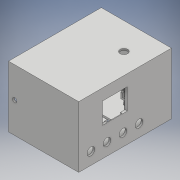
# Autodesk Inventor part: Suporte
Saved by Autodesk Inventor 2018 (Build 220112000, 112)
## iProperties
Created: 2018-04-23
Part Number: Suporte
Material: Genérico
Document SubType Name: Modeling
Designer: mirre
Density: 1 g/cm^3
Appearance: Padrão
Author: mirre
Autodesk Inventor part; units mm, degrees
sketch "Esboço1" plane through (0, 0, 0) normal (0, 0, 1) x (1, 0, 0)
  line L0 (0, 0) -> (118, 0)
  line L1 (118, 0) -> (118, 156)
  line L2 (118, 156) -> (0, 156)
  line L3 (0, 156) -> (0, 0)
  dimension "d0" = 118
  dimension "d1" = 156
  constraints: 8 end point, 2 parallel, 1 horizontal, 1 perpendicular
  measures "d0" distance of L2.end L1.end
  measures "d1" distance of L2.end L0.start
extrude "Extrusão1" add sketch "Esboço1" along normal blind 3
sketch "Esboço2" plane through (0, 0, 3) normal (0, 0, 1) x (1, 0, 0)
  line L0 (3, 3) -> (115, 3)
  line L1 (115, 3) -> (115, 153)
  line L2 (115, 153) -> (3, 153)
  line L3 (3, 153) -> (3, 3)
  line L4 (0, 156) -> (0, 0) projected
  line L5 (118, 156) -> (0, 156) projected
  line L6 (0, 0) -> (118, 0) projected
  line L7 (118, 0) -> (118, 156) projected
  dimension "d4" = 3
  dimension "d5" = 3
  dimension "d6" = 3
  dimension "d7" = 3
  constraints: 8 end point, 2 parallel, 1 horizontal, 1 perpendicular
  measures "d4" distance between parallel lines of L3 L4
  measures "d5" distance between parallel lines of L5 L2
  measures "d6" distance between parallel lines of L6 L0
  measures "d7" distance between parallel lines of L7 L1
extrude "Extrusão2" add sketch "Esboço2" along normal blind 100
sketch "Esboço3" plane through (0, 0, 3) normal (0, 0, 1) x (1, 0, 0)
  line L0 (3, 3) -> (3, 153) projected
  line L1 (3, 3) -> (8, 3)
  line L2 (8, 3) -> (8, 8)
  line L3 (8, 8) -> (3, 8)
  line L4 (3, 8) -> (3, 3)
  line L5 (115, 3) -> (3, 3) projected
  line L6 (68, 3) -> (73, 3)
  line L7 (73, 3) -> (73, 8)
  line L8 (73, 8) -> (68, 8)
  line L9 (68, 8) -> (68, 3)
  line L10 (3, 93) -> (8, 93)
  line L11 (8, 93) -> (8, 98)
  line L12 (8, 98) -> (3, 98)
  line L13 (3, 98) -> (3, 93)
  line L14 (68, 93) -> (73, 93)
  line L15 (73, 93) -> (73, 98)
  line L16 (73, 98) -> (68, 98)
  line L17 (68, 98) -> (68, 93)
  point P0 (0, 0)
  dimension "d10" = 5
  dimension "d11" = 5
  dimension "d12" = 5
  dimension "d13" = 5
  dimension "d14" = 95
  dimension "d15" = 70
  constraints: 32 end point, 8 parallel, 8 point on line, 4 horizontal, 4 perpendicular
  measures "d10" distance of L2.end L3.end
  measures "d11" distance of L7.end L8.end
  measures "d12" distance of L6.end L7.end
  measures "d13" distance of L14.end L15.end
  measures "d14" distance between parallel lines of L12 L1
  measures "d15" distance between parallel lines of L7 L0
extrude "Extrusão3" add sketch "Esboço3" along normal blind 5
sketch "Esboço4" plane through (0, 0, 3) normal (0, 0, 1) x (1, 0, 0)
  line L0 (115, 3) -> (3, 3) projected
  line L1 (3, 3) -> (3, 153) projected
  line L2 (3, 98) -> (23, 98)
  line L3 (23, 98) -> (23, 101)
  line L4 (23, 101) -> (3, 101)
  line L5 (3, 101) -> (3, 98)
  line L6 (73, 3) -> (76, 3)
  line L7 (76, 3) -> (76, 23)
  line L8 (76, 23) -> (73, 23)
  line L9 (73, 23) -> (73, 3)
  line L10 (73, 93) -> (73, 98) projected
  line L11 (73, 98) -> (73, 81)
  line L12 (73, 81) -> (76, 81)
  line L13 (76, 81) -> (76, 101)
  line L14 (76, 101) -> (56, 101)
  line L15 (56, 101) -> (56, 98)
  line L16 (73, 98) -> (68, 98) projected
  line L17 (56, 98) -> (73, 98)
  dimension "d197" = 3
  dimension "d198" = 3
  dimension "d199" = 3
  dimension "d200" = 3
  dimension "d201" = 20
  dimension "d202" = 20
  dimension "d203" = 20
  dimension "d204" = 20
  constraints: 28 end point, 6 perpendicular, 4 parallel, 2 horizontal, 1 collinear, 1 vertical
  measures "d197" distance between parallel lines of L7 L9
  measures "d198" distance between parallel lines of L13 L11
  measures "d199" distance between parallel lines of L14 L17
  measures "d200" distance between parallel lines of L2 L4
  measures "d201" distance between parallel lines of L5 L3
  measures "d202" distance between parallel lines of L13 L15
  measures "d203" distance between parallel lines of L12 L14
  measures "d204" distance between parallel lines of L0 L8
extrude "Extrusão4" add sketch "Esboço4" along normal blind 7
sketch "Esboço5" plane through (118, 0, 0) normal (1, 0, 0) x (0, 0, -1)
  circle A0 centre (-20.5, 20.5) radius 6
  circle A1 centre (-20.5, 47.5) radius 6
  circle A2 centre (-20.5, 74.5) radius 6
  circle A3 centre (-20.5, 101.5) radius 6
  line L0 (-83.5, 40.75) -> (-49, 40.75)
  line L1 (-49, 40.75) -> (-49, 81.25)
  line L2 (-49, 81.25) -> (-83.5, 81.25)
  line L3 (-83.5, 81.25) -> (-83.5, 40.75)
  line L4 (0, 0) -> (0, 156) projected
  line L5 (0, 0) -> (-103, 0) projected
  line L6 (-103, 0) -> (-103, 156) projected
  dimension "d48" = 12
  dimension "d50" = 12
  dimension "d52" = 12
  dimension "d54" = 12
  dimension "d58" = 27
  dimension "d59" = 27
  dimension "d60" = 27
  dimension "d61" = 40.5
  dimension "d62" = 34.5
  dimension "d68" = 20.5
  dimension "d72" = 28.5
  dimension "d73" = 28.5
  dimension "d74" = 28.5
  dimension "d75" = 28.5
  dimension "d76" = 20.5
  dimension "d77" = 20.25
  constraints: 8 end point, 4 centre point, 2 parallel, 1 horizontal, 1 perpendicular
  measures "d48" diameter of A0
  measures "d50" diameter of A1
  measures "d52" diameter of A2
  measures "d54" diameter of A3
  measures "d58" distance of A2.centre A1.centre
  measures "d59" distance of A3.centre A2.centre
  measures "d60" distance of A0.centre A1.centre
  measures "d61" distance between parallel lines of L2 L0
  measures "d62" distance between parallel lines of L1 L3
  measures "d68" distance from line of L5 A0.centre
  measures "d72" distance from line of L1 A0.centre
  measures "d73" distance from line of L1 A1.centre
  measures "d74" distance from line of L1 A2.centre
  measures "d75" distance from line of L1 A3.centre
  measures "d76" distance from line of L4 A3.centre
  measures "d77" distance from line of A3.centre L2
extrude "Extrusão5" cut sketch "Esboço5" against normal blind 20
sketch "Esboço6" plane through (115, 3, 3) normal (-1, 0, 0) x (0, 0, 1)
  line L0 (85.75, 79.5) -> (39.75, 79.5)
  line L1 (39.75, 79.5) -> (39.75, 36.5)
  line L2 (39.75, 36.5) -> (85.75, 36.5)
  line L3 (85.75, 36.5) -> (85.75, 79.5)
  line L4 (-3, -3) -> (100, -3) projected
  line L5 (-3, -3) -> (-3, 153) projected
  line L6 (88.75, 82.5) -> (36.75, 82.5)
  line L7 (36.75, 82.5) -> (36.75, 33.5)
  line L8 (36.75, 33.5) -> (88.75, 33.5)
  line L9 (88.75, 33.5) -> (88.75, 82.5)
  line L10 (46, 37.75) -> (80.5, 37.75) projected
  line L11 (80.5, 37.75) -> (80.5, 78.25) projected
  line L12 (100, -3) -> (100, 153) projected
  dimension "d82" = 1.25
  dimension "d83" = 5.25
  dimension "d84" = 49
  dimension "d85" = 52
  dimension "d88" = 3
  dimension "d89" = 3
  dimension "d90" = 3
  dimension "d91" = 3
  constraints: 16 end point, 4 parallel, 2 horizontal, 2 perpendicular
  measures "d82" distance between parallel lines of L2 L10
  measures "d83" distance between parallel lines of L3 L11
  measures "d84" distance between parallel lines of L8 L6
  measures "d85" distance between parallel lines of L7 L9
  measures "d88" distance between parallel lines of L9 L3
  measures "d89" distance between parallel lines of L8 L2
  measures "d90" distance between parallel lines of L1 L7
  measures "d91" distance between parallel lines of L0 L6
extrude "Extrusão6" add sketch "Esboço6" along normal blind 2.1
sketch "Esboço15" plane through (115, 39.5, 88.75) normal (-1, 0, 0) x (0, 0, 1)
  line L0 (0, 43) -> (-46, 43)
  line L1 (-46, 43) -> (-46, 0)
  line L2 (-46, 0) -> (0, 0)
  line L3 (0, 0) -> (0, 43)
  line L4 (-5.25, 41.75) -> (-39.75, 41.75) projected
  line L5 (-39.75, 1.25) -> (-5.25, 1.25) projected
  line L6 (-39.75, 41.75) -> (-39.75, 1.25) projected
  line L7 (-5.25, 1.25) -> (-5.25, 41.75) projected
  point P0 (-88.75, -39.5)
  dimension "d98" = 1.25
  dimension "d99" = 1.25
  dimension "d100" = 6.25
  dimension "d101" = 5.25
  constraints: 8 end point, 2 parallel, 1 horizontal, 1 perpendicular
  measures "d98" distance between parallel lines of L0 L4
  measures "d99" distance between parallel lines of L2 L5
  measures "d100" distance between parallel lines of L6 L1
  measures "d101" distance between parallel lines of L3 L7
extrude "Extrusão8" add sketch "Esboço15" along normal blind 1
sketch "Esboço17" plane through (114, 39.5, 88.75) normal (-1, 0, 0) x (0, 0, 1)
  line L0 (-4.25, 19.75) -> (2, 19.75)
  line L1 (2, 19.75) -> (2, 36.75)
  line L2 (2, 36.75) -> (-4.25, 36.75)
  line L3 (-4.25, 36.75) -> (-4.25, 19.75)
  line L4 (-40.75, 34.75) -> (-48, 34.75)
  line L5 (-48, 34.75) -> (-48, 8.25)
  line L6 (-48, 8.25) -> (-40.75, 8.25)
  line L7 (-40.75, 8.25) -> (-40.75, 34.75)
  line L8 (3, -3) -> (-49, -3) projected
  line L9 (-49, 46) -> (3, 46) projected
  line L10 (-49, -3) -> (-49, 46) projected
  line L11 (-39.75, 41.75) -> (-39.75, 1.25) projected
  line L12 (-39.75, 1.25) -> (-5.25, 1.25) projected
  line L13 (-5.25, 41.75) -> (-39.75, 41.75) projected
  line L14 (-5.25, 1.25) -> (-5.25, 41.75) projected
  line L15 (3, 46) -> (3, -3) projected
  point P0 (-88.75, -39.5)
  dimension "d108" = 1
  dimension "d109" = 1
  dimension "d110" = 7
  dimension "d111" = 7
  dimension "d112" = 1
  dimension "d113" = 1
  dimension "d114" = 5
  dimension "d115" = 22
  constraints: 16 end point, 4 parallel, 2 horizontal, 2 perpendicular
  measures "d108" distance between parallel lines of L11 L7
  measures "d109" distance between parallel lines of L10 L5
  measures "d110" distance between parallel lines of L12 L6
  measures "d111" distance between parallel lines of L13 L4
  measures "d112" distance between parallel lines of L14 L3
  measures "d113" distance between parallel lines of L15 L1
  measures "d114" distance between parallel lines of L2 L13
  measures "d115" distance between parallel lines of L0 L13
extrude "Extrusão9" cut sketch "Esboço17" against normal blind 3 contours L3 L2 L1 L0 | L7 L6 L5 L4
ref_plane "Plano de trabalho3" through (115, 40.5, 103) normal (-0.9848078, 0, 0.1736482) x (0, -1, 0)
sketch "Esboço30" plane through (115, 40.5, 103) normal (-0.9848078, 0, 0.1736482) x (0, -1, 0)
  line L0 (-106.5, -19.9808) -> (-55, -19.9808)
  line L1 (-55, -19.9808) -> (-55, -63.4808)
  line L2 (-55, -63.4808) -> (-106.5, -63.4808)
  line L3 (-106.5, -63.4808) -> (-106.5, -19.9808)
  line L4 (37.5, -98.4808) -> (-112.5, -98.4808) projected
  line L5 (-45, -11.4437) -> (-45, -62.6538) projected
  point P0 (40.5, -121.4047)
  dimension "d168" = 51.5
  dimension "d169" = 43.5
  dimension "d170" = 35
  dimension "d171" = 10
  constraints: 8 end point, 2 parallel, 1 horizontal, 1 perpendicular
  measures "d168" distance between parallel lines of L1 L3
  measures "d169" distance between parallel lines of L0 L2
  measures "d170" distance between parallel lines of L4 L2
  measures "d171" distance between parallel lines of L5 L1
extrude "Extrusão14" add sketch "Esboço30" along normal up to surface surface through (115, 3, 3) normal (1, 0, 0)
sketch "Esboço32" plane through (115, 40.5, 103) normal (-0.9848078, 0, 0.1736482) x (0.1736482, 0, 0.9848078)
  line L0 (-22.9808, 103.5) -> (-60.4808, 103.5)
  line L1 (-60.4808, 103.5) -> (-60.4808, 58)
  line L2 (-60.4808, 58) -> (-22.9808, 58)
  line L3 (-22.9808, 58) -> (-22.9808, 103.5)
  line L4 (-19.9808, 55) -> (-63.4808, 55) projected
  line L5 (-63.4808, 55) -> (-63.4808, 106.5) projected
  line L6 (-63.4808, 106.5) -> (-19.9808, 106.5) projected
  line L7 (-19.9808, 106.5) -> (-19.9808, 55) projected
  point P0 (-121.4047, -40.5)
  dimension "d174" = 3
  dimension "d175" = 3
  dimension "d176" = 3
  dimension "d177" = 3
  constraints: 8 end point, 2 parallel, 1 horizontal, 1 perpendicular
  measures "d174" distance between parallel lines of L4 L2
  measures "d175" distance between parallel lines of L5 L1
  measures "d176" distance between parallel lines of L6 L0
  measures "d177" distance between parallel lines of L7 L3
ref_plane "Plano de trabalho4" through (117, 0, 0) normal (1, 0, 0) x (0, 0, -1)
extrude "Extrusão15" cut sketch "Esboço32" against normal up to surface contours L3 L2 L1 L0 surface through (117, 0, 0) normal (1, 0, 0)
sketch "Esboço34" plane through (115, 40.5, 103) normal (-0.9848078, 0, 0.1736482) x (0.1736482, 0, 0.9848078)
  line L0 (-63.4808, 106.5) -> (-19.9808, 106.5) projected
  line L1 (-19.9808, 55) -> (-63.4808, 55) projected
  line L2 (-19.9808, 106.5) -> (-63.4808, 106.5)
  line L3 (-63.4808, 106.5) -> (-63.4808, 55)
  line L4 (-63.4808, 55) -> (-19.9808, 55)
  line L5 (-19.9808, 55) -> (-19.9808, 106.5)
  line L6 (-60.4808, 103.5) -> (-60.4808, 58) projected
  line L7 (-22.9808, 103.5) -> (-60.4808, 103.5) projected
  line L8 (-60.4808, 58) -> (-22.9808, 58)
  line L9 (-22.9808, 58) -> (-22.9808, 103.5)
  line L10 (-22.9808, 103.5) -> (-60.4808, 103.5)
  line L11 (-60.4808, 103.5) -> (-60.4808, 58)
  constraints: 16 end point, 4 parallel, 2 horizontal, 2 perpendicular
extrude "Extrusão16" cut sketch "Esboço34" against normal blind 2
ref_plane "Plano de trabalho8" through (115, 75, 82.711) normal (-0.9848078, 0, 0.1736482) x (0, -1, 0)
ref_plane "Plano de trabalho9" through (116.9696, 75, 82.3637) normal (-0.9848078, 0, 0.1736482) x (0, -1, 0)
sketch "Esboço45" plane through (0, 0, 0) normal (-1, 0, 0) x (0, 0, 1)
  circle A0 centre (25, 128) radius 10.05
  line L0 (0, 156) -> (0, 0) projected
  line L1 (0, 156) -> (103, 156) projected
  line L2 (26.25, 140.472) -> (23.75, 140.472)
  line L3 (23.75, 140.472) -> (23.75, 137.972)
  line L4 (26.25, 140.472) -> (26.25, 137.972)
  dimension "d205" = 20.1
  dimension "d206" = 25
  dimension "d207" = 28
  dimension "d210" = 2.5
  dimension "d263" = 2.5
  dimension "d264" = 1.25
  constraints: 6 end point, 2 point on circle, 1 centre point, 1 horizontal, 1 perpendicular, 1 vertical
  measures "d205" diameter of A0
  measures "d206" distance from line of A0.centre L0
  measures "d207" distance from line of L1 A0.centre
  measures "d210" distance of L2.end L3.end
  measures "d263" distance between parallel lines of L4 L3
  measures "d264" distance from line of A0.centre L4
extrude "Extrusão19" cut sketch "Esboço45" against normal blind 10
sketch "Esboço46" plane through (3, 153, 3) normal (0, -1, 0) x (1, 0, 0)
  line L0 (115, 100) -> (-3, 100) projected
  line L1 (115, -3) -> (115, 100) projected
  line L2 (-3, 100) -> (115, 100)
  line L3 (115, 100) -> (115, 97)
  line L4 (115, 97) -> (-3, 97)
  line L5 (-3, 97) -> (-3, 100)
  point P0 (-3, -3)
  dimension "d213" = 3
  constraints: 8 end point, 2 parallel, 1 horizontal, 1 perpendicular, 1 point on line
  measures "d213" distance between parallel lines of L0 L4
extrude "Extrusão20" add sketch "Esboço46" along normal up to surface (150 mm away)
sketch "Esboço48" plane through (0, 0, 103) normal (0, 0, 1) x (1, 0, 0)
  circle A0 centre (83, 111) radius 5.95
  line L0 (118, 156) -> (0, 156) projected
  line L1 (118, 0) -> (118, 156) projected
  point P0 (0, 0)
  dimension "d216" = 11.9
  dimension "d217" = 45
  dimension "d218" = 35
  constraints: 1 centre point
  measures "d216" diameter of A0
  measures "d217" distance from line of L0 A0.centre
  measures "d218" distance from line of L1 A0.centre
extrude "Extrusão21" cut sketch "Esboço48" against normal blind 10
sketch "Esboço49" plane through (0, 0, 0) normal (-1, 0, 0) x (0, 0, 1)
  line L0 (3, 3) -> (3, 153) projected
  line L1 (100, 3) -> (10, 3)
  line L2 (10, 3) -> (10, 100)
  line L3 (10, 100) -> (100, 100)
  line L4 (100, 100) -> (100, 3)
  point P0 (3, 103)
  dimension "d227" = 90
  dimension "d228" = 97
  constraints: 8 end point, 2 parallel, 1 horizontal, 1 perpendicular, 1 point on line
  measures "d227" distance of L2.end L3.end
  measures "d228" distance between parallel lines of L1 L3
extrude "Extrusão22" cut sketch "Esboço49" against normal blind 3
ref_plane "Plano de trabalho10" through (117, 132.625, 79.3121) normal (-0.9848078, 0, 0.1736482) x (0, 1, 0)
sketch "Esboço61" plane through (117, 132.625, 79.3121) normal (-0.9848078, 0, 0.1736482) x (0, 1, 0)
  line L0 (11.375, 37.5) -> (-34.125, 37.5) projected
  line L1 (11.375, 37.5) -> (-34.125, 37.5)
  line L2 (-34.125, 37.5) -> (-34.125, 35.5)
  line L3 (-34.125, 35.5) -> (11.375, 35.5)
  line L4 (11.375, 35.5) -> (11.375, 37.5)
  point P0 (-132.625, 98.424)
  dimension "d267" = 2
  constraints: 8 end point, 2 parallel, 1 horizontal, 1 perpendicular
  measures "d267" distance between parallel lines of L3 L0
extrude "Extrusão27" add sketch "Esboço61" along normal up to surface surface through (117, 121.25, 60.2728) normal (1, 0, 0)
sketch "Esboço62" plane through (0, 156, 0) normal (0, 1, 0) x (1, 0, 0)
  line L0 (63, -62.5) -> (55, -62.5)
  line L1 (55, -62.5) -> (55, -59.5)
  line L2 (55, -59.5) -> (63, -59.5)
  line L3 (63, -59.5) -> (63, -62.5)
  line L4 (0, 0) -> (0, -103) projected
  line L5 (118, 0) -> (0, 0) projected
  dimension "d274" = 8
  dimension "d275" = 3
  dimension "d280" = 59.5
  dimension "d281" = 55
  constraints: 8 end point, 2 parallel, 1 horizontal, 1 perpendicular
  measures "d274" distance between parallel lines of L1 L3
  measures "d275" distance between parallel lines of L0 L2
  measures "d280" distance between parallel lines of L5 L2
  measures "d281" distance between parallel lines of L4 L1
extrude "Extrusão28" cut sketch "Esboço62" against normal blind 10
sketch "Esboço67" plane through (0, 0, 10) normal (0, 0, 1) x (1, 0, 0)
  line L0 (56, 101) -> (76, 101) projected
  line L1 (76, 101) -> (56, 101)
  line L2 (68, 98) -> (56, 98) projected
  line L3 (56, 101) -> (56, 98)
  line L4 (56, 98) -> (68, 98)
  line L5 (68, 93) -> (73, 93) projected
  line L6 (68, 98) -> (68, 93)
  line L7 (68, 93) -> (73, 93)
  line L8 (73, 81) -> (73, 93) projected
  line L9 (73, 93) -> (73, 81)
  line L10 (76, 81) -> (73, 81) projected
  line L11 (73, 81) -> (76, 81)
  line L12 (76, 101) -> (76, 81) projected
  line L13 (76, 81) -> (76, 101)
  line L14 (76, 23) -> (76, 3) projected
  line L15 (76, 23) -> (76, 3)
  line L16 (73, 3) -> (68, 3) projected
  line L17 (76, 3) -> (68, 3)
  line L18 (73, 23) -> (76, 23) projected
  line L19 (76, 23) -> (73, 23)
  line L20 (73, 8) -> (68, 8) projected
  line L21 (73, 23) -> (73, 8)
  line L22 (73, 8) -> (68, 8)
  line L23 (68, 8) -> (68, 3) projected
  line L24 (68, 8) -> (68, 3)
  point P0 (3, 101)
  point P1 (23, 101)
  point P2 (23, 98)
  point P3 (8, 98)
  point P4 (8, 93)
  point P5 (3, 93)
  point P6 (8, 8)
  point P7 (3, 3)
  dimension "d310" = 3
  dimension "d311" = 3
  dimension "d312" = 5
  dimension "d313" = 5
  dimension "d314" = 20
  dimension "d315" = 20
  constraints: 28 end point, 8 collinear, 6 perpendicular
  measures "d310" distance between parallel lines of L12 L8
  measures "d311" distance between parallel lines of L2 L0
  measures "d312" distance between parallel lines of L5 L2
  measures "d313" distance between parallel lines of L8 L6
  measures "d314" distance between parallel lines of L12 L3
  measures "d315" distance between parallel lines of L10 L0
extrude "Extrusão31" cut sketch "Esboço67" against normal blind 10
sketch "Esboço68" plane through (0, 0, 0) normal (-1, 0, 0) x (0, 0, 1)
  line L0 (100, 153) -> (3, 153)
  line L1 (3, 153) -> (3, 3)
  line L2 (3, 3) -> (100, 3)
  line L3 (100, 3) -> (100, 153)
  line L4 (0, 0) -> (103, 0) projected
  line L5 (103, 156) -> (103, 0) projected
  line L6 (0, 156) -> (103, 156) projected
  line L7 (0, 156) -> (0, 0) projected
  dimension "d318" = 3
  dimension "d319" = 3
  dimension "d320" = 3
  dimension "d321" = 3
  constraints: 8 end point, 2 parallel, 1 horizontal, 1 perpendicular
  measures "d318" distance between parallel lines of L4 L2
  measures "d319" distance between parallel lines of L5 L3
  measures "d320" distance between parallel lines of L6 L0
  measures "d321" distance between parallel lines of L7 L1
extrude "Extrusão32" cut sketch "Esboço68" against normal blind 3 contours L3 L2 L1 L0
sketch "Esboço76" plane through (0, 0, 10) normal (0, 0, 1) x (1, 0, 0)
  line L0 (3, 3) -> (3, 8) projected
  line L1 (8, 8) -> (3, 8) projected
  line L2 (3, 3) -> (8, 3)
  line L3 (8, 3) -> (8, 8)
  line L4 (8, 8) -> (3, 8)
  line L5 (3, 8) -> (3, 3)
  line L6 (23, 101) -> (23, 98) projected
  line L7 (3, 101) -> (23, 101) projected
  line L8 (23, 101) -> (3, 101)
  line L9 (3, 93) -> (3, 98) projected
  line L10 (3, 101) -> (3, 93)
  line L11 (3, 93) -> (8, 93) projected
  line L12 (3, 93) -> (8, 93)
  line L13 (8, 98) -> (8, 93) projected
  line L14 (8, 93) -> (8, 98)
  line L15 (23, 98) -> (8, 98) projected
  line L16 (8, 98) -> (23, 98)
  line L17 (23, 98) -> (23, 101)
  constraints: 20 end point, 3 collinear, 3 perpendicular, 2 horizontal, 2 parallel
extrude "Extrusão33" cut sketch "Esboço76" against normal up to surface (7 mm away)
sketch "Esboço77" plane through (0, 0, 0) normal (0, -1, 0) x (1, 0, 0)
  circle A0 centre (10.5, 51.5) radius 3.55
  line L0 (0, 103) -> (118, 103) projected
  line L1 (0, 0) -> (0, 103) projected
  dimension "d332" = 7.1
  dimension "d333" = 51.5
  dimension "d334" = 10.5
  constraints: 1 centre point
  measures "d332" diameter of A0
  measures "d333" distance from line of L0 A0.centre
  measures "d334" distance from line of L1 A0.centre
extrude "Extrusão34" cut sketch "Esboço77" against normal through all
sketch "Esboço80" plane through (0, 156, 0) normal (0, 1, 0) x (1, 0, 0)
  line L0 (0, 0) -> (0, -103) projected
  line L1 (0, -9) -> (4, -9)
  line L2 (4, -9) -> (4, -7)
  line L3 (4, -7) -> (0, -7)
  line L4 (0, -7) -> (0, -9)
  line L5 (118, 0) -> (0, 0) projected
  dimension "d340" = 2
  dimension "d341" = 4
  dimension "d342" = 7
  constraints: 8 end point, 2 parallel, 1 horizontal, 1 perpendicular, 1 point on line
  measures "d340" distance between parallel lines of L1 L3
  measures "d341" distance between parallel lines of L0 L2
  measures "d342" distance between parallel lines of L5 L3
extrude "Extrusão35" cut sketch "Esboço80" against normal blind 10
ref_plane "Plano de trabalho11" through (117, 132.625, 79.3121) normal (-0.9848078, 0, 0.1736482) x (0, 1, 0)
sketch "Esboço82" plane through (117, 132.625, 79.3121) normal (-0.9848078, 0, 0.1736482) x (0, 1, 0)
  line L0 (14.375, -3) -> (-37.125, -3)
  line L1 (-37.125, -3) -> (-37.125, 40.5)
  line L2 (-37.125, 40.5) -> (14.375, 40.5)
  line L3 (14.375, 40.5) -> (14.375, -3)
  line L4 (-34.125, 37.5) -> (11.375, 37.5)
  line L5 (11.375, 37.5) -> (11.375, 0)
  line L6 (11.375, 0) -> (-34.125, 0)
  line L7 (-34.125, 0) -> (-34.125, 37.5)
  point P0 (-132.625, 98.424)
  point P1 (14.375, 40.5)
  dimension "d346" = 43.5
  dimension "d347" = 51.5
  dimension "d348" = 3
  dimension "d349" = 3
  dimension "d350" = 3
  dimension "d351" = 3
  constraints: 16 end point, 4 parallel, 2 horizontal, 2 perpendicular
  measures "d346" distance between parallel lines of L2 L0
  measures "d347" distance between parallel lines of L3 L1
  measures "d348" distance between parallel lines of L1 L7
  measures "d349" distance between parallel lines of L0 L6
  measures "d350" distance between parallel lines of L5 L3
  measures "d351" distance between parallel lines of L2 L4
extrude "Extrusão36" add sketch "Esboço82" along normal blind 12.2
sketch "Esboço84" plane through (112.9, 3, 3) normal (-1, 0, 0) x (0, 0, 1)
  line L0 (36.75, 82.5) -> (88.75, 82.5) projected
  line L1 (88.75, 33.5) -> (36.75, 33.5) projected
  line L2 (88.75, 82.5) -> (36.75, 82.5)
  line L3 (36.75, 82.5) -> (36.75, 33.5)
  line L4 (36.75, 33.5) -> (88.75, 33.5)
  line L5 (88.75, 33.5) -> (88.75, 82.5)
  line L6 (39.75, 79.5) -> (85.75, 79.5) projected
  line L7 (39.75, 36.5) -> (39.75, 79.5) projected
  line L8 (85.75, 79.5) -> (39.75, 79.5)
  line L9 (39.75, 79.5) -> (39.75, 36.5)
  line L10 (39.75, 36.5) -> (85.75, 36.5)
  line L11 (85.75, 36.5) -> (85.75, 79.5)
  point P0 (-3, -3)
  constraints: 16 end point, 4 parallel, 2 horizontal, 2 perpendicular
extrude "Extrusão37" add sketch "Esboço84" along normal blind 1
sketch "Esboço85" plane through (115, 36.5, 39.75) normal (0, -1, 0) x (1, 0, 0)
  line L0 (-3.1, 49) -> (-3.1, 3) projected
  line L1 (-3.1, 20) -> (-9.1, 20)
  line L2 (-9.1, 20) -> (-9.1, 30)
  line L3 (-9.1, 30) -> (-6.1, 30)
  line L4 (-6.1, 30) -> (-6.1, 23)
  line L5 (-6.1, 23) -> (-3.1, 23)
  line L6 (-3.1, 23) -> (-3.1, 20)
  line L7 (0, 0) -> (-3.1, 0) projected
  point P0 (-115, -39.75)
  dimension "d356" = 6
  dimension "d357" = 3
  dimension "d358" = 3
  dimension "d359" = 10
  dimension "d360" = 20
  constraints: 12 end point, 5 perpendicular, 2 point on line, 1 horizontal
  measures "d356" distance between parallel lines of L0 L2
  measures "d357" distance between parallel lines of L0 L4
  measures "d358" distance between parallel lines of L1 L5
  measures "d359" distance between parallel lines of L3 L1
  measures "d360" distance between parallel lines of L7 L1
extrude "Extrusão38" add sketch "Esboço85" against normal blind 3
sketch "Esboço86" plane through (114, 82.5, 42.75) normal (0, -1, 0) x (1, 0, 0)
  line L0 (-8.1, 27) -> (-5.1, 27)
  line L1 (-5.1, 27) -> (-5.1, 20)
  line L2 (-5.1, 20) -> (-2.1, 20)
  line L3 (-2.1, 49) -> (-2.1, -3) projected
  line L4 (-2.1, 20) -> (-2.1, 17)
  line L5 (-8.1, 17) -> (-8.1, 27)
  line L6 (-8.1, 17) -> (-2.1, 17)
  line L7 (1, -3) -> (-2.1, -3) projected
  point P0 (-114, -42.75)
  dimension "d363" = 20
  dimension "d364" = 10
  dimension "d365" = 6
  dimension "d366" = 3
  dimension "d367" = 3
  constraints: 12 end point, 2 horizontal, 2 perpendicular, 2 point on line, 1 parallel
  measures "d363" distance between parallel lines of L7 L6
  measures "d364" distance between parallel lines of L0 L6
  measures "d365" distance between parallel lines of L3 L5
  measures "d366" distance between parallel lines of L3 L1
  measures "d367" distance between parallel lines of L2 L6
extrude "Extrusão39" add sketch "Esboço86" against normal blind 3
sketch "Esboço89" plane through (115, 95.5, 38.5399) normal (0, -1, 0) x (1, 0, 0)
  line L0 (-9.4937, 45.8451) -> (-17.0474, 3.0059) projected
  line L1 (-14.4427, 17.778) -> (-20.3515, 18.8199)
  line L2 (-20.3515, 18.8199) -> (-18.615, 28.668)
  line L3 (-18.615, 28.668) -> (-15.6606, 28.1471)
  line L4 (-15.6606, 28.1471) -> (-16.8762, 21.2534)
  line L5 (-16.8762, 21.2534) -> (-13.9217, 20.7325)
  line L6 (-13.9217, 20.7325) -> (-14.4427, 17.778)
  line L7 (-17.0474, 3.0059) -> (0, 0) projected
  point P0 (-115, -38.5399)
  dimension "d370" = 6
  dimension "d371" = 3
  dimension "d372" = 15
  dimension "d373" = 10
  dimension "d374" = 3
  constraints: 12 end point, 3 parallel, 2 perpendicular, 2 point on line
  measures "d370" distance between parallel lines of L2 L0
  measures "d371" distance between parallel lines of L0 L4
  measures "d372" distance between parallel lines of L7 L1
  measures "d373" distance between parallel lines of L1 L3
  measures "d374" distance between parallel lines of L1 L5
extrude "Extrusão40" add sketch "Esboço89" against normal blind 3
sketch "Esboço90" plane through (117, 144, 43.2644) normal (0, -1, 0) x (1, 0, 0)
  line L0 (-22.3515, 14.0954) -> (-16.4427, 13.0536)
  line L1 (-11.4937, 41.1206) -> (-19.0474, -1.7186) projected
  line L2 (-16.4427, 13.0536) -> (-15.9217, 16.008)
  line L3 (-15.9217, 16.008) -> (-18.8762, 16.5289)
  line L4 (-18.8762, 16.5289) -> (-17.6606, 23.4226)
  line L5 (-17.6606, 23.4226) -> (-20.615, 23.9435)
  line L6 (-19.0474, -1.7186) -> (-2, -4.7245) projected
  line L7 (-20.615, 23.9435) -> (-22.3515, 14.0954)
  point P0 (-117, -43.2644)
  dimension "d377" = 15
  dimension "d378" = 10
  dimension "d379" = 3
  dimension "d380" = 6
  dimension "d381" = 3
  constraints: 12 end point, 3 perpendicular, 2 parallel, 1 collinear, 1 point on line
  measures "d377" distance between parallel lines of L6 L0
  measures "d378" distance between parallel lines of L5 L0
  measures "d379" distance between parallel lines of L0 L3
  measures "d380" distance between parallel lines of L1 L7
  measures "d381" distance between parallel lines of L1 L4
extrude "Extrusão41" add sketch "Esboço90" against normal blind 3
sketch "Esboço98" plane through (0, 156, 0) normal (0, 1, 0) x (1, 0, 0)
  line L0 (70, -54.5) -> (48, -54.5)
  line L1 (48, -54.5) -> (48, -22)
  line L2 (48, -22) -> (70, -22)
  line L3 (70, -22) -> (70, -54.5)
  line L4 (55, -59.5) -> (63, -59.5) projected
  line L5 (0, -9) -> (0, -103) projected
  circle A0 centre (65.5, -45) radius 1.75
  circle A1 centre (52.5, -45) radius 1.75
  point P0 (0, 0)
  dimension "d385" = 22
  dimension "d386" = 32.5
  dimension "d387" = 5
  dimension "d388" = 48
  dimension "d390" = 3.5
  dimension "d391" = 9.5
  dimension "d392" = 9.5
  dimension "d393" = 4.5
  dimension "d394" = 4.5
  dimension "d401" = 3.5
  constraints: 8 end point, 2 centre point, 2 parallel, 1 horizontal, 1 perpendicular
  measures "d385" distance of L1.end L2.end
  measures "d386" distance between parallel lines of L0 L2
  measures "d387" distance between parallel lines of L4 L0
  measures "d388" distance between parallel lines of L5 L1
  measures "d390" diameter of A0
  measures "d391" distance from line of L0 A1.centre
  measures "d392" distance from line of L0 A0.centre
  measures "d393" distance from line of L1 A1.centre
  measures "d394" distance from line of L3 A0.centre
  measures "d401" diameter of A1
extrude "Extrusão42" cut sketch "Esboço98" against normal blind 10 contours A0 | A1
sketch "Esboço99" plane through (0, 156, 0) normal (0, 1, 0) x (1, 0, 0)
  line L0 (70, -54.5) -> (48, -54.5)
  line L1 (48, -54.5) -> (48, -22)
  line L2 (48, -22) -> (70, -22)
  line L3 (70, -22) -> (70, -54.5)
  line L4 (55, -59.5) -> (63, -59.5) projected
  line L5 (0, -9) -> (0, -103) projected
  line L6 (64.5, -41.5) -> (53.5, -41.5)
  line L7 (53.5, -41.5) -> (53.5, -37.5)
  line L8 (53.5, -37.5) -> (64.5, -37.5)
  line L9 (64.5, -37.5) -> (64.5, -41.5)
  point P0 (0, 0)
  dimension "d415" = 22
  dimension "d416" = 32.5
  dimension "d417" = 5
  dimension "d418" = 48
  dimension "d419" = 11
  dimension "d421" = 16.5
  dimension "d423" = 4
  dimension "d424" = 17
  constraints: 16 end point, 4 parallel, 2 horizontal, 2 perpendicular
  measures "d415" distance of L1.end L2.end
  measures "d416" distance of L2.end L0.start
  measures "d417" distance between parallel lines of L4 L0
  measures "d418" distance between parallel lines of L5 L1
  measures "d419" distance of L8.end L7.end
  measures "d421" distance between parallel lines of L1 L9
  measures "d423" distance between parallel lines of L6 L8
  measures "d424" distance between parallel lines of L0 L8
extrude "Extrusão43" cut sketch "Esboço99" against normal blind 2 contours L6 L7 L8 L9
sketch "Esboço101" plane through (0, 156, 0) normal (0, 1, 0) x (1, 0, 0)
  circle A0 centre (10.5, -51.5) radius 3.55 projected
  circle A1 centre (10.5, -51.5) radius 3.75
  point P0 (0, 0)
  dimension "d427" = 7.5
  constraints: 1 centre point, 1 coincident
  measures "d427" diameter of A1
extrude "Extrusão44" cut sketch "Esboço101" against normal through all
sketch "Esboço102" plane through (0, 156, 0) normal (0, 1, 0) x (1, 0, 0)
  line L0 (63.5, -63) -> (54.5, -63)
  line L1 (54.5, -63) -> (54.5, -59)
  line L2 (54.5, -59) -> (63.5, -59)
  line L3 (63.5, -59) -> (63.5, -63)
  line L4 (63, -62.5) -> (55, -62.5) projected
  line L5 (55, -59.5) -> (63, -59.5) projected
  line L6 (55, -62.5) -> (55, -59.5) projected
  line L7 (63, -59.5) -> (63, -62.5) projected
  dimension "d430" = 0.5
  dimension "d431" = 0.5
  dimension "d432" = 0.5
  dimension "d433" = 0.5
  constraints: 8 end point, 2 parallel, 1 horizontal, 1 perpendicular
  measures "d430" distance between parallel lines of L0 L4
  measures "d431" distance between parallel lines of L2 L5
  measures "d432" distance between parallel lines of L1 L6
  measures "d433" distance between parallel lines of L3 L7
extrude "Extrusão47" cut sketch "Esboço102" against normal blind 10
sketch "Esboço103" plane through (0, 156, 0) normal (0, 1, 0) x (1, 0, 0)
  line L0 (65, -42) -> (53, -42)
  line L1 (53, -42) -> (53, -37)
  line L2 (53, -37) -> (65, -37)
  line L3 (65, -37) -> (65, -42)
  line L4 (53.5, -41.5) -> (53.5, -37.5) projected
  line L5 (53.5, -37.5) -> (64.5, -37.5) projected
  line L6 (64.5, -37.5) -> (64.5, -41.5) projected
  line L7 (64.5, -41.5) -> (53.5, -41.5) projected
  point P0 (0, 0)
  dimension "d444" = 0.5
  dimension "d445" = 0.5
  dimension "d446" = 0.5
  dimension "d447" = 0.5
  constraints: 8 end point, 2 parallel, 1 horizontal, 1 perpendicular
  measures "d444" distance between parallel lines of L1 L4
  measures "d445" distance between parallel lines of L5 L2
  measures "d446" distance between parallel lines of L3 L6
  measures "d447" distance between parallel lines of L0 L7
extrude "Extrusão48" cut sketch "Esboço103" against normal up to surface (2 mm away)
sketch "Esboço104" plane through (0, 156, 0) normal (0, 1, 0) x (1, 0, 0)
  line L0 (4, -9) -> (0, -9) projected
  line L1 (4, -9) -> (4.5, -9)
  line L2 (4.5, -9) -> (4.5, -7)
  line L3 (4.5, -7) -> (4, -7)
  line L4 (4, -7) -> (4, -9)
  line L5 (0, -7) -> (4, -7) projected
  point P0 (0, 0)
  dimension "d450" = 0.5
  constraints: 8 end point, 2 parallel, 1 collinear, 1 horizontal, 1 perpendicular
  measures "d450" distance of L3.end L2.end
extrude "Extrusão49" cut sketch "Esboço104" against normal blind 10
sketch "Esboço105" plane through (118, 0, 0) normal (1, 0, 0) x (0, 0, -1)
  circle A0 centre (-20.5, 20.5) radius 6 projected
  circle A1 centre (-20.5, 20.5) radius 6.5
  circle A2 centre (-20.5, 47.5) radius 6.5
  circle A3 centre (-20.5, 74.5) radius 6.5
  circle A4 centre (-20.5, 101.5) radius 6.5
  circle A5 centre (-20.5, 101.5) radius 6 projected
  circle A6 centre (-20.5, 74.5) radius 6 projected
  circle A7 centre (-20.5, 47.5) radius 6 projected
  circle A8 centre (-20.5, 20.5) radius 6 projected
  point P0 (0, 0)
  dimension "d453" = 13
  dimension "d454" = 13
  dimension "d455" = 13
  dimension "d456" = 13
  constraints: 4 centre point, 4 concentric, 1 coincident
  measures "d453" diameter of A1
  measures "d454" diameter of A2
  measures "d455" diameter of A3
  measures "d456" diameter of A4
extrude "Extrusão50" cut sketch "Esboço105" against normal blind 10 contours A0 | A1 | A2 | A3 | A4 | A5 | A6 | A7
sketch "Esboço107" plane through (0, 0, 103) normal (0, 0, 1) x (1, 0, 0)
  circle A0 centre (83, 111) radius 5.95 projected
  circle A1 centre (83, 111) radius 6.45
  point P0 (0, 0)
  dimension "d459" = 12.9
  constraints: 1 centre point, 1 coincident
  measures "d459" diameter of A1
extrude "Extrusão51" cut sketch "Esboço107" against normal blind 10
sketch "Esboço108" plane through (0, 0, 0) normal (0, 0, -1) x (-1, 0, 0)
  line L0 (-55.9, 101.1) -> (-76.1, 101.1)
  line L1 (-76.1, 101.1) -> (-76.1, 80.9)
  line L2 (-76.1, 80.9) -> (-72.9, 80.9)
  line L3 (-72.9, 80.9) -> (-72.9, 92.9)
  line L4 (-72.9, 92.9) -> (-67.9, 92.9)
  line L5 (-67.9, 92.9) -> (-67.9, 97.9)
  line L6 (-67.9, 97.9) -> (-55.9, 97.9)
  line L7 (-55.9, 97.9) -> (-55.9, 101.1)
  line L8 (-72.9, 23.1) -> (-76.1, 23.1)
  line L9 (-76.1, 23.1) -> (-76.1, 2.9)
  line L10 (-76.1, 2.9) -> (-67.9, 2.9)
  line L11 (-67.9, 2.9) -> (-67.9, 8.1)
  line L12 (-72.9, 23.1) -> (-72.9, 8.1)
  line L13 (-72.9, 8.1) -> (-67.9, 8.1)
  line L14 (-73, 93) -> (-73, 81) projected
  line L15 (-73, 81) -> (-76, 81) projected
  line L16 (-76, 81) -> (-76, 101) projected
  line L17 (-76, 101) -> (-56, 101) projected
  line L18 (-56, 101) -> (-56, 98) projected
  line L19 (-56, 98) -> (-68, 98) projected
  line L20 (-68, 98) -> (-68, 93) projected
  line L21 (-68, 93) -> (-73, 93) projected
  line L22 (-68, 3) -> (-76, 3) projected
  line L23 (-76, 23) -> (-73, 23) projected
  line L24 (-76, 3) -> (-76, 23) projected
  line L25 (-73, 23) -> (-73, 8) projected
  line L26 (-73, 8) -> (-68, 8) projected
  line L27 (-68, 8) -> (-68, 3) projected
  point P0 (0, 0)
  dimension "d462" = 0.1
  dimension "d463" = 0.1
  dimension "d464" = 0.1
  dimension "d465" = 0.1
  dimension "d466" = 0.1
  dimension "d467" = 0.1
  dimension "d468" = 0.1
  dimension "d469" = 0.1
  dimension "d470" = 0.1
  dimension "d471" = 0.1
  dimension "d472" = 0.1
  dimension "d473" = 0.1
  dimension "d474" = 0.1
  dimension "d475" = 0.1
  constraints: 28 end point, 11 perpendicular, 2 horizontal, 1 vertical
  measures "d462" distance between parallel lines of L3 L14
  measures "d463" distance between parallel lines of L2 L15
  measures "d464" distance between parallel lines of L16 L1
  measures "d465" distance between parallel lines of L17 L0
  measures "d466" distance between parallel lines of L7 L18
  measures "d467" distance between parallel lines of L6 L19
  measures "d468" distance between parallel lines of L20 L5
  measures "d469" distance between parallel lines of L21 L4
  measures "d470" distance between parallel lines of L10 L22
  measures "d471" distance between parallel lines of L8 L23
  measures "d472" distance between parallel lines of L24 L9
  measures "d473" distance between parallel lines of L12 L25
  measures "d474" distance between parallel lines of L26 L13
  measures "d475" distance between parallel lines of L11 L27
extrude "Extrusão52" cut sketch "Esboço108" against normal blind 10 contours L7 L6 L5 L4 L3 L2 L1 L0 | L12 L13 L11 L10 L9 L8 | L14 L15 L16 L17 L18 L19 L20 L21 | L22 L24 L23 L25 L26 L27
sketch "Esboço114" plane through (114, 39.5, 88.75) normal (-1, 0, 0) x (0, 0, 1)
  line L0 (-48, 8.25) -> (-48, 34.75) projected
  line L1 (-40.75, 8.25) -> (-48, 8.25) projected
  line L2 (-48, 34.75) -> (-46, 34.75)
  line L3 (-46, 34.75) -> (-46, 8.25)
  line L4 (-46, 8.25) -> (-48, 8.25)
  line L5 (-48, 8.25) -> (-48, 34.75)
  line L6 (-46, 0) -> (-46, 43) projected
  line L7 (-4.25, 36.75) -> (2, 36.75) projected
  line L8 (2, 36.75) -> (0, 36.75)
  line L9 (0, 36.75) -> (0, 19.6977)
  line L10 (0, 19.6977) -> (2, 19.6977)
  line L11 (2, 19.6977) -> (2, 36.75)
  line L12 (0, 43) -> (0, 0) projected
  point P0 (-88.75, -39.5)
  constraints: 16 end point, 4 parallel, 2 collinear, 2 horizontal, 2 perpendicular, 1 point on line
extrude "Extrusão56" add sketch "Esboço114" against normal up to surface (3 mm away)
sketch "Esboço115" plane through (114, 39.5, 88.75) normal (-1, 0, 0) x (0, 0, 1)
  line L0 (-4.75, 42.25) -> (-40.25, 42.25)
  line L1 (-40.25, 42.25) -> (-40.25, 0.75)
  line L2 (-40.25, 0.75) -> (-4.75, 0.75)
  line L3 (-4.75, 0.75) -> (-4.75, 42.25)
  line L4 (-39.75, 1.25) -> (-5.25, 1.25) projected
  line L5 (-5.25, 1.25) -> (-5.25, 41.75) projected
  line L6 (-5.25, 41.75) -> (-39.75, 41.75) projected
  line L7 (-39.75, 41.75) -> (-39.75, 1.25) projected
  line L8 (-39.75, 1.25) -> (-39.75, 41.75) projected
  line L9 (-5.25, 41.75) -> (-39.75, 41.75)
  line L10 (-39.75, 41.75) -> (-39.75, 1.25)
  line L11 (-39.75, 1.25) -> (-5.25, 1.25)
  line L12 (-5.25, 1.25) -> (-5.25, 41.75)
  point P0 (-88.75, -39.5)
  dimension "d497" = 0.5
  dimension "d498" = 0.5
  dimension "d499" = 0.5
  dimension "d500" = 0.5
  constraints: 16 end point, 4 parallel, 2 horizontal, 2 perpendicular
  measures "d497" distance between parallel lines of L2 L4
  measures "d498" distance between parallel lines of L3 L5
  measures "d499" distance between parallel lines of L6 L0
  measures "d500" distance between parallel lines of L7 L1
extrude "Extrusão57" cut sketch "Esboço115" against normal blind 10
sketch "Esboço116" plane through (111.9, 3, 3) normal (-1, 0, 0) x (0, 0, 1)
  line L0 (86.25, 80) -> (39.25, 80)
  line L1 (39.25, 80) -> (39.25, 36)
  line L2 (39.25, 36) -> (86.25, 36)
  line L3 (86.25, 36) -> (86.25, 80)
  line L4 (85.75, 79.5) -> (85.75, 36.5) projected
  line L5 (39.75, 36.5) -> (39.75, 79.5) projected
  line L6 (85.75, 36.5) -> (59.75, 36.5) projected
  line L7 (59.75, 79.5) -> (85.75, 79.5) projected
  line L8 (85.75, 36.5) -> (39.75, 36.5) projected
  line L9 (85.75, 79.5) -> (39.75, 79.5)
  line L10 (39.75, 79.5) -> (39.75, 36.5)
  line L11 (39.75, 36.5) -> (85.75, 36.5)
  line L12 (85.75, 36.5) -> (85.75, 79.5)
  point P0 (-3, -3)
  dimension "d503" = 0.5
  dimension "d504" = 0.5
  dimension "d505" = 0.5
  dimension "d506" = 0.5
  constraints: 16 end point, 4 parallel, 2 horizontal, 2 perpendicular
  measures "d503" distance between parallel lines of L3 L4
  measures "d504" distance between parallel lines of L5 L1
  measures "d505" distance between parallel lines of L2 L6
  measures "d506" distance between parallel lines of L7 L0
extrude "Extrusão58" cut sketch "Esboço116" against normal up to surface (2.1 mm away)
sketch "Esboço117" plane through (114, 39.5, 88.75) normal (-1, 0, 0) x (0, 0, 1)
  line L0 (-4.75, 42.25) -> (-4.75, 0.75) projected
  line L1 (0.5, 43.5) -> (0.5, -0.5) projected
  line L2 (-4.75, 36.75) -> (0.5, 36.75)
  line L3 (0.5, 36.75) -> (0.5, 19.75)
  line L4 (0.5, 19.75) -> (-4.75, 19.75)
  line L5 (-4.75, 19.75) -> (-4.75, 36.75)
  line L6 (0, 19.75) -> (-4.25, 19.75) projected
  line L7 (-4.25, 36.75) -> (0, 36.75) projected
  line L8 (-46.5, -0.5) -> (-46.5, 43.5) projected
  line L9 (-40.25, 34.75) -> (-46.5, 34.75)
  line L10 (-46.5, 34.75) -> (-46.5, 8.25)
  line L11 (-46.5, 8.25) -> (-40.25, 8.25)
  line L12 (-40.25, 8.25) -> (-40.25, 34.75)
  line L13 (-46, 34.75) -> (-40.75, 34.75) projected
  line L14 (-40.75, 8.25) -> (-46, 8.25) projected
  line L15 (-40.25, 0.75) -> (-40.25, 42.25) projected
  point P0 (-88.75, -39.5)
  constraints: 16 end point, 5 collinear, 4 parallel, 3 point on line, 2 horizontal, 2 perpendicular
extrude "Extrusão59" cut sketch "Esboço117" against normal up to surface (3 mm away)
sketch "Esboço119" plane through (115, 3, 3) normal (-1, 0, 0) x (0, 0, 1)
  line L0 (89.25, 83) -> (36.25, 83)
  line L1 (36.25, 83) -> (36.25, 33)
  line L2 (36.25, 33) -> (89.25, 33)
  line L3 (89.25, 33) -> (89.25, 83)
  line L4 (88.75, 33.5) -> (88.75, 82.5) projected
  line L5 (36.75, 82.5) -> (36.75, 33.5) projected
  line L6 (59.75, 33.5) -> (88.75, 33.5) projected
  line L7 (88.75, 82.5) -> (59.75, 82.5) projected
  line L8 (88.75, 82.5) -> (88.75, 33.5) projected
  line L9 (88.75, 82.5) -> (36.75, 82.5)
  line L10 (36.75, 82.5) -> (36.75, 33.5)
  line L11 (36.75, 33.5) -> (88.75, 33.5)
  line L12 (88.75, 33.5) -> (88.75, 82.5)
  point P0 (-3, -3)
  dimension "d515" = 0.5
  dimension "d516" = 0.5
  dimension "d517" = 0.5
  dimension "d518" = 0.5
  constraints: 16 end point, 4 parallel, 2 horizontal, 2 perpendicular
  measures "d515" distance between parallel lines of L3 L4
  measures "d516" distance between parallel lines of L1 L5
  measures "d517" distance between parallel lines of L2 L6
  measures "d518" distance between parallel lines of L7 L0
extrude "Extrusão60" add sketch "Esboço119" along normal up to surface (3.1 mm away)
sketch "Esboço120" plane through (105.9, 85.5, 59.75) normal (0, 1, 0) x (1, 0, 0)
  line L0 (0, 0) -> (6, 0) projected
  line L1 (6, 0) -> (0, 0)
  line L2 (0, 0) -> (0, -10)
  line L3 (3, -10) -> (0, -10) projected
  line L4 (0, -10) -> (3, -10)
  line L5 (3, -10) -> (3, -3)
  line L6 (6, -3) -> (3, -3) projected
  line L7 (3, -3) -> (6, -3)
  line L8 (6, -3) -> (6, 0)
  point P0 (-105.9, 59.75)
  constraints: 12 end point, 3 collinear, 3 perpendicular
extrude "Extrusão61" add sketch "Esboço120" along normal blind 0.5
sketch "Esboço121" plane through (105.9, 36.5, 59.75) normal (0, -1, 0) x (1, 0, 0)
  line L0 (6, 3) -> (6, 32.5) projected
  line L1 (3, 3) -> (6, 3) projected
  line L2 (6, 3) -> (3, 3)
  line L3 (0, 10) -> (3, 10) projected
  line L4 (3, 3) -> (3, 10)
  line L5 (3, 10) -> (0, 10)
  line L6 (0, 10) -> (0, 0)
  line L7 (6, 0) -> (0, 0) projected
  line L8 (0, 0) -> (6, 0)
  line L9 (6, -17.5) -> (6, 0) projected
  line L10 (6, 0) -> (6, 3)
  point P0 (-105.9, -59.75)
  constraints: 12 end point, 4 collinear, 2 perpendicular
extrude "Extrusão62" add sketch "Esboço121" along normal blind 0.5
sketch "Esboço122" plane through (111.9, 3, 3) normal (1, 0, 0) x (0, 0, -1)
  line L0 (-66.75, 36) -> (-56.75, 36)
  line L1 (-56.75, 36) -> (-56.75, 80)
  line L2 (-56.75, 80) -> (-66.75, 80)
  line L3 (-66.75, 80) -> (-66.75, 36)
  line L4 (-66.75, 79.5) -> (-66.75, 83) projected
  line L5 (-56.75, 36.5) -> (-56.75, 33) projected
  line L6 (-66.75, 36.5) -> (-59.75, 36.5) projected
  line L7 (-59.75, 79.5) -> (-66.75, 79.5) projected
  point P0 (3, -3)
  dimension "d525" = 0.5
  dimension "d526" = 0.5
  constraints: 8 end point, 2 collinear, 2 parallel, 1 horizontal, 1 perpendicular
  measures "d525" distance between parallel lines of L6 L0
  measures "d526" distance between parallel lines of L7 L2
extrude "Extrusão63" cut sketch "Esboço122" against normal blind 10
sketch "Esboço124" plane through (104.9853, 132.625, 81.4306) normal (-0.9848078, 0, 0.1736482) x (0.1736482, 0, 0.9848078)
  line L0 (3.5, 14.875) -> (-41, 14.875)
  line L1 (-41, 14.875) -> (-41, -37.625)
  line L2 (-41, -37.625) -> (3.5, -37.625)
  line L3 (3.5, -37.625) -> (3.5, 14.875)
  line L4 (3, -37.125) -> (-40.5, -37.125) projected
  line L5 (3, 14.375) -> (3, -37.125) projected
  line L6 (-40.5, 14.375) -> (3, 14.375) projected
  line L7 (-40.5, -37.125) -> (-40.5, 14.375) projected
  line L8 (3, 14.375) -> (-40.5, 14.375)
  line L9 (-40.5, 14.375) -> (-40.5, -37.125)
  line L10 (-40.5, -37.125) -> (3, -37.125)
  line L11 (3, -37.125) -> (3, 14.375)
  point P0 (-98.424, -132.625)
  dimension "d529" = 0.5
  dimension "d530" = 0.5
  dimension "d531" = 0.5
  dimension "d532" = 0.5
  constraints: 16 end point, 4 parallel, 2 horizontal, 2 perpendicular
  measures "d529" distance between parallel lines of L2 L4
  measures "d530" distance between parallel lines of L3 L5
  measures "d531" distance between parallel lines of L6 L0
  measures "d532" distance between parallel lines of L1 L7
extrude "Extrusão64" add sketch "Esboço124" against normal up to surface surface through (115, 3, 3) normal (1, 0, 0)
sketch "Esboço125" plane through (104.9853, 132.625, 81.4306) normal (-0.9848078, 0, 0.1736482) x (0.1736482, 0, 0.9848078)
  line L0 (0.5, 11.875) -> (-38, 11.875)
  line L1 (-38, 11.875) -> (-38, -34.625)
  line L2 (-38, -34.625) -> (0.5, -34.625)
  line L3 (0.5, -34.625) -> (0.5, 11.875)
  line L4 (-35.5, -34.125) -> (0, -34.125) projected
  line L5 (0, -34.125) -> (0, 11.375) projected
  line L6 (0, 11.375) -> (-35.5, 11.375) projected
  line L7 (-37.5, -34.125) -> (-37.5, 11.375) projected
  line L8 (0, 11.375) -> (-37.5, 11.375)
  line L9 (-37.5, 11.375) -> (-37.5, -34.125)
  line L10 (-37.5, -34.125) -> (0, -34.125)
  line L11 (0, -34.125) -> (0, 11.375)
  point P0 (-98.424, -132.625)
  dimension "d535" = 0.5
  dimension "d536" = 0.5
  dimension "d537" = 0.5
  dimension "d538" = 0.5
  constraints: 16 end point, 4 parallel, 2 horizontal, 2 perpendicular
  measures "d535" distance between parallel lines of L2 L4
  measures "d536" distance between parallel lines of L3 L5
  measures "d537" distance between parallel lines of L6 L0
  measures "d538" distance between parallel lines of L7 L1
extrude "Extrusão65" cut sketch "Esboço125" against normal up to surface surface through (117, 121.25, 60.2728) normal (1, 0, 0)
sketch "Esboço127" plane through (117, 132.625, 79.3121) normal (-0.9848078, 0, 0.1736482) x (0.1736482, 0, 0.9848078)
  line L0 (0.5, 11.875) -> (-38, 11.875) projected
  line L1 (-38, 11.875) -> (-38, -34.625) projected
  line L2 (-36, 11.875) -> (-38, 11.875)
  line L3 (-38, 11.875) -> (-38, -34.625)
  line L4 (-38, -34.625) -> (-36, -34.625)
  line L5 (-36, -34.625) -> (-36, 11.875)
  dimension "d541" = 2
  constraints: 8 end point, 2 parallel, 1 horizontal, 1 perpendicular, 1 point on line
  measures "d541" distance between parallel lines of L5 L1
extrude "Extrusão66" add sketch "Esboço127" along normal up to surface surface through (117, 121.25, 60.2728) normal (1, 0, 0)
sketch "Esboço128" plane through (117, 132.625, 79.3121) normal (-0.9848078, 0, 0.1736482) x (0.1736482, 0, 0.9848078)
  line L0 (-35.5, -34.125) -> (-35.5, 11.375) projected
  line L1 (-35.5, 11.375) -> (-36, 11.375)
  line L2 (-36, 11.375) -> (-36, -34.125)
  line L3 (-36, -34.125) -> (-35.5, -34.125)
  line L4 (-35.5, -34.125) -> (-35.5, 11.375)
  line L5 (-36, 11.375) -> (-36, 11.875) projected
  constraints: 8 end point, 2 parallel, 1 collinear, 1 horizontal, 1 perpendicular
extrude "Extrusão67" cut sketch "Esboço128" along normal up to surface surface through (117, 121.25, 60.2728) normal (1, 0, 0)
sketch "Esboço129" plane through (96.385, 147, 67.2079) normal (0, 1, 0) x (0.9848078, 0, -0.1736482)
  line L0 (6, 10) -> (6, 7) projected
  line L1 (6, 10) -> (6, 7)
  line L2 (3, 0) -> (3, 7) projected
  line L3 (6, 7) -> (3, 7)
  line L4 (3, 7) -> (3, 0)
  line L5 (0, 0) -> (3, 0) projected
  line L6 (3, 0) -> (0, 0)
  line L7 (0, 10) -> (0, 0) projected
  line L8 (0, 0) -> (0, 10)
  line L9 (0, 10) -> (6, 10) projected
  line L10 (0, 10) -> (6, 10)
  point P0 (-83.2501, 82.924)
  constraints: 12 end point, 4 perpendicular, 2 collinear
extrude "Extrusão68" add sketch "Esboço129" along normal blind 0.5 and the other way blind 52
sketch "Esboço130" plane through (96.385, 95, 67.2079) normal (-0.9848078, 0, 0.1736482) x (0.1736482, 0, 0.9848078)
  line L0 (0, 0) -> (0, 52.5) projected
  line L1 (-10, 0) -> (-10, 3) projected
  line L2 (0, 49.5) -> (-10, 49.5)
  line L3 (-10, 49.5) -> (-10, 3)
  line L4 (-10, 3) -> (0, 3)
  line L5 (0, 3) -> (0, 49.5)
  line L6 (-7, 49.5) -> (16, 49.5) projected
  line L7 (16, 3) -> (-7, 3) projected
  point P0 (-82.924, -95)
  constraints: 8 end point, 2 collinear, 2 parallel, 2 point on line, 1 horizontal, 1 perpendicular
extrude "Extrusão69" cut sketch "Esboço130" against normal up to surface surface through (117, 121.25, 60.2728) normal (1, 0, 0)
sketch "Esboço131" plane through (0, 156, 0) normal (0, 1, 0) x (1, 0, 0)
  circle A0 centre (20, -20) radius 10.3
  line L0 (30.1902, -18.5) -> (32.6902, -18.5)
  line L1 (32.6902, -18.5) -> (32.6902, -21.5)
  line L2 (32.6902, -21.5) -> (30.1902, -21.5)
  line L3 (0, -9) -> (0, -103) projected
  line L4 (118, 0) -> (0, 0) projected
  dimension "d552" = 20.6
  dimension "d553" = 3
  dimension "d554" = 1.5
  dimension "d555" = 2.5
  dimension "d556" = 20
  dimension "d557" = 20
  constraints: 6 end point, 2 perpendicular, 2 point on circle, 1 centre point, 1 horizontal
  measures "d552" diameter of A0
  measures "d553" distance between parallel lines of L0 L2
  measures "d554" distance from line of A0.centre L2
  measures "d555" distance of L0.start L0.end
  measures "d556" distance from line of L3 A0.centre
  measures "d557" distance from line of A0.centre L4
extrude "Extrusão70" cut sketch "Esboço131" against normal blind 3
